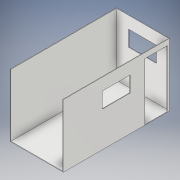
# Autodesk Inventor part: Koffer_leer
Saved by Autodesk Inventor 2018 (Build 220112000, 112)
## iProperties
Created: 2020-03-17
Part Number: Koffer_leer
Material: Generisch
Document SubType Name: Modeling
Designer: wepet
Density: 1 g/cm^3
Appearance: Vorgabe
Author: wepet
Autodesk Inventor part; units mm, degrees
ref_plane "YZ Plane" through (0, 0, 0) normal (1, 0, 0) x (0, 1, 0)
ref_plane "XZ Plane" through (0, 0, 0) normal (0, 1, 0) x (-1, 0, 0)
ref_plane "XY Plane" through (0, 0, 0) normal (0, 0, 1) x (1, 0, 0)
sketch "Skizze1" plane through (0, 0, 0) normal (0, 0, 1) x (1, 0, 0)
  line L0 (-76.5, 0) -> (76.5, 0)
  line L1 (76.5, 0) -> (76.5, 306.5)
  line L2 (76.5, 306.5) -> (-76.5, 306.5)
  line L3 (-76.5, 306.5) -> (-76.5, 0)
  line L4 (75, 306.5) -> (75, 0) construction
  line L5 (-75, 0) -> (-75, 306.5) construction
  line L6 (-76.5, 305) -> (76.5, 305) construction
  point P0 (0, 0)
  point P1 (0, 0)
  point P2 (-75, 305)
  point P3 (75, 305)
  dimension "d2" = 1.5
  dimension "d3" = 1.5
  dimension "d4" = 1.5
  dimension "d5" = 150
  dimension "d6" = 305
  constraints: 14 end point, 10 point on line, 4 perpendicular, 2 parallel, 1 coincident, 1 horizontal, 1 midpoint
  measures "d2" distance between parallel lines of L4 L1
  measures "d3" distance between parallel lines of L3 L5
  measures "d4" distance between parallel lines of L2 L6
  measures "d5" distance between parallel lines of L4 L5
  measures "d6" distance between parallel lines of L0 L6
extrude "Bodenplatte" add sketch "Skizze1" along normal blind 1.8
sketch "Skizze3" plane through (0, 0, 1.8) normal (0, 0, 1) x (1, 0, 0)
  line L0 (-76.5, 306.5) -> (-76.5, 0) projected
  line L1 (-76.5, 0) -> (76.5, 0) projected
  line L2 (-76.5, 306.5) -> (-75, 306.5)
  line L3 (-75, 306.5) -> (-75, 0)
  line L4 (-75, 0) -> (-76.5, 0)
  line L5 (-76.5, 0) -> (-76.5, 306.5)
  point P0 (0, 0)
  dimension "d9" = 1.5
  constraints: 8 end point, 2 parallel, 1 horizontal, 1 perpendicular, 1 point on line
  measures "d9" distance between parallel lines of L0 L3
extrude "Wand_links" add sketch "Skizze3" along normal blind 180
sketch "Skizze4" plane through (0, 0, 1.8) normal (0, 0, 1) x (1, 0, 0)
  line L0 (76.5, 0) -> (76.5, 306.5) projected
  line L1 (76.5, 0) -> (75, 0)
  line L2 (75, 0) -> (75, 306.5)
  line L3 (75, 306.5) -> (76.5, 306.5)
  line L4 (76.5, 306.5) -> (76.5, 0)
  point P0 (0, 0)
  dimension "d12" = 1.5
  constraints: 8 end point, 2 parallel, 1 horizontal, 1 perpendicular
  measures "d12" distance between parallel lines of L0 L2
extrude "Wand_rechts" add sketch "Skizze4" along normal blind 180
sketch "Skizze5" plane through (0, 0, 1.8) normal (0, 0, 1) x (1, 0, 0)
  line L0 (75, 306.5) -> (-75, 306.5) projected
  line L1 (75, 306.5) -> (75, 0) projected
  line L2 (-75, 0) -> (-75, 306.5) projected
  line L3 (-75, 306.5) -> (-76.5, 306.5) projected
  line L4 (-75, 306.5) -> (75, 306.5)
  line L5 (75, 306.5) -> (75, 305)
  line L6 (75, 305) -> (-75, 305)
  line L7 (-75, 305) -> (-75, 306.5)
  point P0 (0, 0)
  dimension "d15" = 1.5
  constraints: 8 end point, 2 parallel, 1 horizontal, 1 perpendicular, 1 point on line
  measures "d15" distance between parallel lines of L6 L0
extrude "Wand_vorn" add sketch "Skizze5" along normal blind 180
sketch "Skizze6" plane through (-76.5, 306.5, 0) normal (0, 1, 0) x (1, 0, 0)
  line L0 (153, 0) -> (0, 0) construction
  line L1 (0, 0) -> (0, -181.8) construction
  line L2 (153, -181.8) -> (0, -181.8) construction
  line L3 (153, 0) -> (153, -181.8) construction
  line L4 (115.5, -147.2) -> (37.5, -147.2)
  line L5 (36.3, -146) -> (36.3, -103)
  line L6 (37.5, -101.8) -> (115.5, -101.8)
  line L7 (116.7, -103) -> (116.7, -146)
  line L8 (76.5, 0) -> (76.5, -181.8) construction
  line L9 (153, 0) -> (153, -181.8) construction
  line L10 (151.5, -1.8) -> (1.5, -1.8) construction
  arc A0 (115.5, -147.2) -> (116.7, -146) centre (115.5, -146) ccw
  arc A1 (36.3, -146) -> (37.5, -147.2) centre (37.5, -146) ccw
  arc A2 (37.5, -101.8) -> (36.3, -103) centre (37.5, -103) ccw
  arc A3 (116.7, -103) -> (115.5, -101.8) centre (115.5, -103) ccw
  point P0 (116.7, -147.2)
  point P1 (36.3, -101.8)
  point P2 (36.3, -147.2)
  point P3 (116.7, -101.8)
  point P4 (76.5, -147.2)
  dimension "d18" = 80.4
  dimension "d19" = 45.4
  dimension "d25" = 100
  dimension "d35" = 1.2
  constraints: 10 end point, 9 point on line, 8 point on circle, 8 tangent, 4 centre point, 3 equal radius, 2 midpoint, 2 parallel, 1 horizontal, 1 perpendicular
  measures "d18" distance of point (36.3, -101.8) point (116.7, -101.8)
  measures "d19" distance of point (36.3, -147.2) point (36.3, -101.8)
  measures "d25" distance between parallel lines of L6 L10
  measures "d35" radius of A0
extrude "Fenster_vorn" cut sketch "Skizze6" against normal up to next
sketch "Skizze7" plane through (76.5, 0, 0) normal (1, 0, 0) x (0, 0, -1)
  line L0 (-1.8, 0) -> (-1.8, 305) construction
  line L1 (-181.8, 305) -> (-1.8, 305) construction
  line L2 (-146, 112.3) -> (-103, 112.3)
  line L3 (-101.8, 113.5) -> (-101.8, 191.5)
  line L4 (-103, 192.7) -> (-146, 192.7)
  line L5 (-147.2, 191.5) -> (-147.2, 113.5)
  arc A0 (-147.2, 113.5) -> (-146, 112.3) centre (-146, 113.5) ccw
  arc A1 (-146, 192.7) -> (-147.2, 191.5) centre (-146, 191.5) ccw
  arc A2 (-101.8, 191.5) -> (-103, 192.7) centre (-103, 191.5) ccw
  arc A3 (-103, 112.3) -> (-101.8, 113.5) centre (-103, 113.5) ccw
  line L6 (-1.8, 152.5) -> (-181.8, 152.5) construction
  line L7 (-181.8, 0) -> (-181.8, 305) construction
  point P0 (0, 0)
  point P1 (-101.8, 192.7)
  point P2 (-101.8, 112.3)
  point P3 (-147.2, 192.7)
  point P4 (-147.2, 152.5)
  dimension "d26" = 45.4
  dimension "d27" = 80.4
  dimension "d28" = 1.2
  dimension "d29" = 1.2
  dimension "d30" = 1.2
  dimension "d31" = 1.2
  dimension "d34" = 100
  constraints: 10 end point, 8 point on circle, 8 tangent, 7 point on line, 4 centre point, 3 midpoint, 2 parallel, 1 horizontal, 1 perpendicular
  measures "d26" distance of point (-147.2, 192.7) point (-101.8, 192.7)
  measures "d27" distance of point (-101.8, 192.7) point (-101.8, 112.3)
  measures "d28" radius of A0
  measures "d29" radius of A1
  measures "d30" radius of A2
  measures "d31" radius of A3
  measures "d34" distance between parallel lines of L0 L3
extrude "Fenster_rechts" cut sketch "Skizze7" against normal blind 10
sketch "Skizze8" plane through (76.5, 0, 0) normal (1, 0, 0) x (0, 0, -1)
  line L0 (-181.8, 305) -> (-1.8, 305) construction
  line L1 (-1.8, 0) -> (-1.8, 305) construction
  line L2 (-166.8, 235) -> (-1.8, 235)
  line L3 (-1.8, 235) -> (-1.8, 300)
  line L4 (-1.8, 300) -> (-166.8, 300)
  line L5 (-166.8, 300) -> (-166.8, 235)
  point P0 (0, 0)
  dimension "d36" = 65
  dimension "d37" = 165
  dimension "d38" = 5
  constraints: 8 end point, 2 parallel, 1 collinear, 1 horizontal, 1 perpendicular
  measures "d36" distance of L4.end L2.start
  measures "d37" distance of L3.end L4.end
  measures "d38" distance between parallel lines of L0 L4
extrude "Tuer_rechts" cut sketch "Skizze8" against normal blind 10
